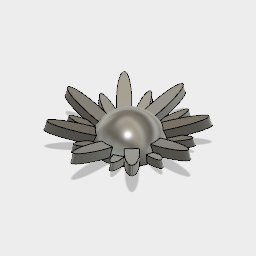
花 (Autodesk Fusion 360 design; units mm, degrees)
Autodesk Fusion 360 part; units mm, degrees
sketch "草图1" plane through (0, 0, 0) normal (0, 1, 0) x (1, 0, 0)
  ellipse E0 centre (20, -15) end of major axis (30, -15) minor radius 2
extrude "拉伸1" add sketch "草图1" along normal blind 3 makes body 1
move_body "移动1" bodies 1 to x (0.965926, 0.258819, 0) y (-0.258819, 0.965926, 0) z (0, 0, 1) at (0.3407, -2.5882, 0)
box "长方体基本要素1" add length 6 width 6 height 6 placed x (0, -1, 0) y (1, 0, 0) z (0, 0, 1) at (-8, 2, 0) separate body makes body 2
move_body "移动2" bodies 2 to x (1, 0, 0) y (0, 1, 0) z (0, 0, 1) at (9.4721, 4.0516, 0)
move_body "移动3" bodies 2 to x (1, 0, 0) y (0, 1, 0) z (0, 0, 1) at (0, 0, 10)
pattern_circular "C-阵列1" count 8 over 360 about axis through (7.4721, 0.0516, 16) along (0, 1, 0) of bodies 1 makes body 3 at (12.8266, 3.1853, 6.4317) makes body 4 at (4.563, 2.7827, 6.9506) makes body 5 at (-0.7963, 3.747, 11.8452) makes body 6 at (-1.3185, 3.7486, 18.9091) makes body 7 at (3.3172, 3.747, 24.2684) makes body 8 at (10.3812, 3.7486, 24.7906) makes body 9 at (17.0403, 3.1853, 21.3545)
copy_body "复制和粘贴实体1" bodies 4 5 3 6 7 8 9 1 makes body 10 makes body 11 makes body 12 makes body 13 makes body 14 makes body 15 makes body 16 makes body 17
move_body "移动4" bodies 10 11 12 13 14 15 16 17 to x (1, 0, 0) y (0, 1, 0) z (0, 0, 1) at (0, -152.6303, -181.9765)
scale "缩放1" factor 0.8 about (8.4721, -149.7325, -164.225) bodies 14 13 17 12 10 16 15 11
move_body "移动5" bodies 15 10 12 17 16 14 11 13 to x (1, 0, 0) y (0, 1, 0) z (0, 0, 1) at (0, 150, 180)
move_body "移动6" bodies 15 2 11 12 16 13 14 17 10 to x (0.906308, 0, -0.422618) y (0, 1, 0) z (0.422618, 0, 0.906308) at (-6.0618, 0, 4.6569)
sphere "球体基本要素1" add diameter 20 placed x (1, 0, 0) y (0, 0, -1) z (0, 1, 0) at (42, 0, 12) separate body makes body 18
move_body "MoveFace1" bodies 18 to x (1, 0, 0) y (0, 1, 0) z (0, 0, 1) at (-33, 0, 3) on bodies 18
move_body "移动7" bodies 18 to x (1, 0, 0) y (0, 1, 0) z (0, 0, 1) at (-1, 0, 1)
combine "合并1" operation add target body 1 tool bodies 17 3 4 5 6 7 8 9 10 11 12 13 14 15 16 18
box "长方体基本要素2" add length 60 width 60 height 40 placed x (0, 0, 1) y (1, 0, 0) z (0, 1, 0) at (16, 0, 48) separate body makes body 19
move_body "移动8" bodies 19 to x (1, 0, 0) y (0, 1, 0) z (0, 0, 1) at (-40, -40, -60)
combine "合并2" operation cut target body 1 tool bodies 19
hidden bodies 2
